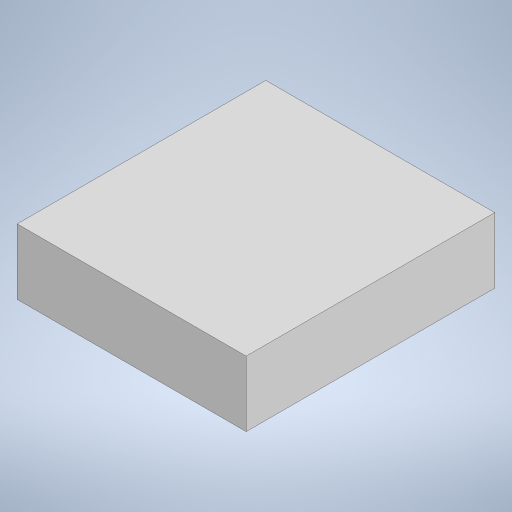
# Autodesk Inventor part: meinnkibann
Saved by Autodesk Inventor 2023 (Build 270158000, 158)
## iProperties
Created: 2022-09-27
Part Number: meinnkibann
Material: 一般
Document SubType Name: Modeling
Designer: ellie
Density: 1 g/cm^3
Appearance: 既定
Author: ellie
Autodesk Inventor part; units mm, degrees
ref_plane "YZ Plane" through (0, 0, 0) normal (1, 0, 0) x (0, 1, 0)
ref_plane "XZ Plane" through (0, 0, 0) normal (0, 1, 0) x (-1, 0, 0)
ref_plane "XY Plane" through (0, 0, 0) normal (0, 0, 1) x (1, 0, 0)
sketch "スケッチ1" plane through (0, 0, 0) normal (0, 1, 0) x (-1, 0, 0)
  line L0 (17.736, 19) -> (-17.264, 19)
  line L1 (-17.264, 19) -> (-17.264, -19)
  line L2 (-17.264, -19) -> (17.736, -19)
  line L3 (17.736, -19) -> (17.736, 19)
  line L4 (17.736, 19) -> (-17.264, -19) construction
  line L5 (-17.264, 19) -> (17.736, -19) construction
  point P0 (0, 0)
  point P1 (0.236, 0)
  dimension "d0" = 35
  dimension "d1" = 38
  dimension "d2" = 17.264
  dimension "d3" = 19
  constraints: 12 end point, 2 midpoint, 2 parallel, 1 horizontal, 1 perpendicular
  measures "d0" distance of L2.end L1.end
  measures "d1" distance of L1.end L0.end
  measures "d2" horizontal distance of L1.end point (0, 0)
  measures "d3" vertical distance of L0.start point (0, 0)
extrude "押し出し1" add sketch "スケッチ1" along normal blind 10
